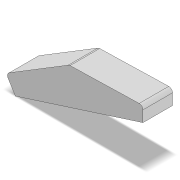
# Autodesk Inventor part: Part2
Saved by Autodesk Inventor 2020 (Build 240168000, 168)
## iProperties
Created: 2019-07-08
Part Number: Part2
Material: Generic
Document SubType Name: Modeling
Designer: chitl
Density: 1 g/cm^3
Appearance: Default
Author: chitl
Autodesk Inventor part; units mm, degrees
ref_plane "YZ Plane" through (0, 0, 0) normal (1, 0, 0) x (0, 1, 0)
ref_plane "XZ Plane" through (0, 0, 0) normal (0, 1, 0) x (-1, 0, 0)
ref_plane "XY Plane" through (0, 0, 0) normal (0, 0, 1) x (1, 0, 0)
sketch "Sketch1" plane through (0, 0, 0) normal (0, 0, 1) x (1, 0, 0)
  line L0 (-54.1531, -3.8255) -> (0, 29.3361)
  line L1 (0, 29.3361) -> (63.5, 30.9789)
  line L2 (-54.1531, -3.8255) -> (-46.1859, -16.836)
  line L3 (-46.1859, -16.836) -> (63.5, 18.2222)
  line L4 (63.5, 18.2222) -> (63.5, 30.9789)
  point P0 (0, 0)
  dimension "d0" = 150
  dimension "d1" = 63.5
  dimension "d2" = 63.5
  constraints: 10 end point, 1 vertical
  measures "d0" angle of L0 L1
  measures "d1" horizontal distance of L0.end L1.end
  measures "d2" distance of L0.start L0.end
extrude "Extrusion1" add sketch "Sketch1" along normal blind 25.4
fillet "Fillet1" radius 3.175 1 edges at (0, 29.3361, 12.7)
fillet "Fillet2" radius 3.175 1 edges at (63.5, 30.9789, 12.7)
fillet "Fillet3" radius 3.175 1 edges at (-54.1531, -3.8255, 12.7)
sketch "Sketch2" plane through (63.5, 18.2222, 0) normal (0.3045, -0.9525, 0) x (0.9525, 0.3045, 0)
  line L0 (-105.1746, 19.5706) -> (-8.2146, 19.5706)
  line L1 (-8.2146, 19.5706) -> (-8.2146, 4.4663)
  line L2 (-8.2146, 4.4663) -> (-105.1746, 4.4663)
  line L3 (-105.1746, 4.4663) -> (-105.1746, 19.5706)
  point P0 (-66.0333, 0)
  constraints: 8 end point, 2 parallel, 1 horizontal, 1 perpendicular
extrude "Extrusion2" cut sketch "Sketch2" against normal blind 11.1125
body "Solid1"
